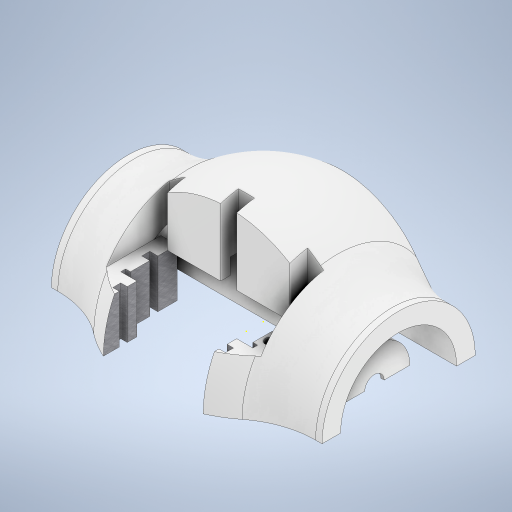
# Autodesk Inventor part: back moter middle lemon printing
Saved by Autodesk Inventor 2023 (Build 270158000, 158)
## iProperties
Created: 2022-10-08
Part Number: back moter middle lemon printing
Material: ABS プラスチック
Document SubType Name: Modeling
Designer: ellie
Density: 1.06 g/cm^3
Appearance: 積雪
Author: ellie
Autodesk Inventor part; units mm, degrees
ref_plane "YZ Plane" through (0, 0, 0) normal (1, 0, 0) x (0, 1, 0)
ref_plane "XZ Plane" through (0, 0, 0) normal (0, 1, 0) x (-1, 0, 0)
ref_plane "XY Plane" through (0, 0, 0) normal (0, 0, 1) x (1, 0, 0)
sketch "スケッチ1" plane through (0, 0, 0) normal (0, 1, 0) x (-1, 0, 0)
  circle A0 centre (0, 0) radius 37.5
  line L0 (0, 0) -> (0, -37.5)
  line L1 (0, 0) -> (0, 37.5)
  dimension "d0" = 75
  constraints: 4 end point, 2 point on circle, 2 vertical, 1 centre point, 1 coincident
  measures "d0" diameter of A0
revolve "回転1" add sketch "スケッチ1" angle 180 about axis through (0, 0, 0) along (0, 0, 1) picked at (-2.7815, -24.6866) contours L1 L0 A0
sketch "スケッチ5" plane through (0, 0, 0) normal (0, -1, 0) x (1, 0, 0)
  line L0 (-21, -21) -> (21, -21)
  line L1 (21, -21) -> (21, -9)
  line L2 (21, -9) -> (-21, -9)
  line L3 (-21, -9) -> (-21, -21)
  line L4 (-21, -11) -> (-21, -9)
  line L5 (0, 29.25) -> (-17.5, 29.25)
  line L6 (-17.5, 29.25) -> (-17.5, 26.75)
  line L7 (-17.5, 26.75) -> (0, 26.75)
  line L8 (0, 26.75) -> (0, 29.25)
  line L9 (0, 23.75) -> (-20.5, 23.75)
  line L10 (-20.5, 23.75) -> (-20.5, 22.25)
  line L11 (-20.5, 22.25) -> (0, 22.25)
  line L12 (0, 22.25) -> (0, 23.75)
  line L13 (0, 16.25) -> (-21.5, 16.25)
  line L14 (-21.5, 16.25) -> (-21.5, 13.75)
  line L15 (-21.5, 13.75) -> (0, 13.75)
  line L16 (0, 13.75) -> (0, 16.25)
  line L17 (0, 7.75) -> (-24, 7.75)
  line L18 (-24, 7.75) -> (-24, 5.25)
  line L19 (-24, 5.25) -> (0, 5.25)
  line L20 (0, 5.25) -> (0, 7.75)
  circle A0 centre (0, 0) radius 37.5 projected
  circle A1 centre (0, 0) radius 37.5 projected
  line L21 (0, 37.5) -> (0, -37.5)
  line L22 (37.5, 0) -> (-37.5, 0)
  line L23 (-33.5, 5.25) -> (-24, 5.25)
  line L24 (-24, 5.25) -> (-24, -5.25)
  line L25 (-24, -5.25) -> (-33.5, -5.25)
  line L26 (-33.5, -5.25) -> (-33.5, 5.25)
  line L27 (-24, -8.0262) -> (-24, 5.25)
  line L28 (-29, 23.775) -> (-29, -23.775)
  line L29 (-15.5, 29.25) -> (0, 29.25)
  line L30 (0, 29.25) -> (0, 37.5)
  line L31 (0, 37.5) -> (-15.5, 37.5)
  line L32 (-15.5, 37.5) -> (-15.5, 29.25)
  line L33 (-15.5, 26.75) -> (0, 26.75)
  line L34 (0, 26.75) -> (0, 23.75)
  line L35 (0, 23.75) -> (-15.5, 23.75)
  line L36 (-15.5, 23.75) -> (-15.5, 26.75)
  line L37 (-19, 16.25) -> (0, 16.25)
  line L38 (0, 16.25) -> (0, 22.25)
  line L39 (0, 22.25) -> (-19, 22.25)
  line L40 (-19, 22.25) -> (-19, 16.25)
  line L41 (-19, 13.75) -> (0, 13.75)
  line L42 (0, 13.75) -> (0, 7.75)
  line L43 (0, 7.75) -> (-19, 7.75)
  line L44 (-19, 7.75) -> (-19, 13.75)
  line L45 (-24, 0) -> (-40.9365, 0)
  line L46 (-24, 0) -> (-9.0837, 0)
  line L47 (-8.5, 5.25) -> (-24, 5.25)
  line L48 (-24, 5.25) -> (-24, -5.25)
  line L49 (-24, -5.25) -> (-8.5, -5.25)
  line L50 (-8.5, 5.25) -> (-24, -5.25) construction
  line L51 (-24, 5.25) -> (-8.5, -5.25) construction
  line L52 (-24, 7.25) -> (-34.5, 7.25)
  line L53 (-34.5, 7.25) -> (-34.5, -7.25)
  line L54 (-34.5, -7.25) -> (-24, -7.25)
  line L55 (-24, -7.25) -> (-24, 7.25)
  line L56 (-24, 7.25) -> (-34.5, -7.25) construction
  line L57 (-34.5, 7.25) -> (-24, -7.25) construction
  line L58 (-8.5, 5.25) -> (-1, 5.25)
  line L59 (-1, 5.25) -> (-1, -5.25)
  line L60 (-1, -5.25) -> (-8.5, -5.25)
  line L61 (-8.5, 5.25) -> (-1, -5.25) construction
  line L62 (-1, 5.25) -> (-8.5, -5.25) construction
  line L63 (-24, 5.25) -> (-29, 5.25)
  line L64 (-24, -5.25) -> (-29, -5.25)
  line L65 (-24, 7.25) -> (-29, 7.25)
  line L66 (-24, -7.25) -> (-29, -7.25)
  line L67 (28.3901, -24.5) -> (-28.3901, -24.5)
  line L68 (-8.5, 5.25) -> (-7.3, 5.25)
  line L69 (-7.3, -5.25) -> (-8.5, -5.25)
  line L70 (-4, 7.75) -> (-1, 7.75)
  line L71 (0, 23.75) -> (-4, 23.75)
  line L72 (-4, 22.25) -> (0, 22.25)
  line L73 (0, 22.25) -> (0, 23.75)
  line L74 (-7, 7.75) -> (-2, 7.75)
  line L75 (-1, 5.25) -> (-6.5, 5.25)
  point P0 (0, -21)
  point P1 (0, -9)
  point P2 (0, 28)
  point P3 (0, 23)
  point P4 (0, 15)
  point P5 (0, 6.5)
  point P6 (-21, -15)
  point P7 (-27, -0.5262)
  point P8 (-15.5, 25.25)
  point P9 (-15.5, 34.1467)
  point P10 (0, 29.25)
  point P11 (0, 26.75)
  point P12 (0, 13.75)
  point P13 (0, 16.25)
  point P14 (-29, 0)
  point P15 (-33.5, 0)
  point P16 (-24, 0)
  point P17 (-16.25, 0)
  point P18 (-29.25, 0)
  point P19 (-4.75, 0)
  point P20 (-27, 0.5)
  point P21 (-28, 0.4738)
  point P22 (-28, -11.5262)
  point P23 (-27, -11.5)
  point P24 (-24, 5.25)
  point P25 (-24, 5.25)
  point P26 (-24, 5.25)
  point P27 (-1, 0)
  point P28 (28.3901, -24.5)
  point P29 (-28.3901, -24.5)
  point P30 (0, 22.25)
  point P31 (0, 23.75)
  point P32 (-29, -7.25)
  point P33 (-29, 7.25)
  point P34 (-7.9, -5.25)
  point P35 (-7.9, 5.25)
  dimension "d12" = 42
  dimension "d13" = 12
  dimension "d23" = 17.5
  dimension "d24" = 2.5
  dimension "d27" = 20.5
  dimension "d28" = 1.5
  dimension "d30" = 21.5
  dimension "d31" = 2.5
  dimension "d33" = 2.5
  dimension "d88" = 0
  dimension "d89" = 0
  dimension "d90" = 16.5
  dimension "d92" = 21
  dimension "d97" = 9.5
  dimension "d98" = 10.5
  dimension "d113" = 29
  dimension "d122" = 15.5
  dimension "d124" = 3
  dimension "d125" = 15.5
  dimension "d126" = 6
  dimension "d127" = 6
  dimension "d128" = 19
  dimension "d129" = 19
  dimension "d161" = 14.5
  dimension "d162" = 10.5
  dimension "d164" = 10.5
  dimension "d170" = 24.5
  dimension "d326" = 23
  dimension "d327" = 10.5
  dimension "d329" = 15.5
  dimension "d330" = 34.5
  dimension "d357" = 8.25
  constraints: 150 end point, 28 parallel, 21 horizontal, 17 midpoint, 16 perpendicular, 16 point on line, 10 collinear, 1 tangent, 1 vertical, 20 other
  measures "d12" distance of L2.end L1.end
  measures "d13" distance of L1.end L0.end
  measures "d23" distance of L7.end L6.end
  measures "d24" distance of L6.end L5.end
  measures "d27" distance of L11.end L10.end
  measures "d28" distance of L10.end L9.end
  measures "d30" distance of L15.end L14.end
  measures "d31" distance of L14.end L13.end
  measures "d33" distance of L18.end L17.end
  measures "d89" distance from line of point (0, 0) L22
  measures "d90" distance from line of L0 point (0, -37.5)
  measures "d92" distance of the line from the sketch origin of L3
  measures "d97" distance of L24.end L25.end
  measures "d98" distance of L23.end L24.end
  measures "d113" distance of the line from the sketch origin of L28
  measures "d122" distance of the line from the sketch origin of L32
  measures "d124" distance of L33.end L34.end
  measures "d126" distance of L38.end L37.end
  measures "d127" distance of L41.end L42.end
  measures "d128" distance of the line from the sketch origin of L44
  measures "d129" distance of the line from the sketch origin of L40
  measures "d161" distance between parallel lines of L54 L52
  measures "d162" distance between parallel lines of L48 L53
  measures "d164" distance between parallel lines of L60 L58
  measures "d170" distance between parallel lines of L67 L22
  measures "d326" distance between parallel lines of L48 L59
  measures "d327" distance between parallel lines of L49 L47
  measures "d329" distance of L48.end L49.end
  measures "d330" distance of the line from the sketch origin of L53
  measures "d357" distance between parallel lines of L5 L31
extrude "GNSボード" cut sketch "スケッチ5" against normal blind 16 contours L8 L7 L6 L5
extrude "GNSボード止めるよう" cut sketch "スケッチ5" against normal blind 15 contours L21 L5 L32 A0 | L21 L9 L36 L7
extrude "アルミ板１" cut sketch "スケッチ5" against normal blind 20 contours L11 L10 L9 L12
extrude "メイン基板" cut sketch "スケッチ5" against normal blind 21 contours L15 L14 L13 L16
extrude "メイン止めるよう" cut sketch "スケッチ5" against normal blind 15 contours L17 L44 L15 L21 | L13 L40 L11 L21
extrude "アルミ板２" cut sketch "スケッチ5" against normal blind 20 contours L19 L18 L17 L20
extrude "電池ボックス入れ" cut sketch "スケッチ5" against normal blind 13 contours L3 L2 L21 L0 | L21 L2 L1 L0
extrude "side ut" cut sketch "スケッチ5" against normal blind 100 contours A0 L22 L53 L54 L28 | A0 L28 L52 L53 L22 | L54 L53 L22 L26 L25 L28 | L53 L52 L28 L23 L26 L22 | L25 L26 L22 L28 | L22 L26 L23 L28
extrude "motor case" add sketch "スケッチ5" against normal blind 7 contours L54 L53 L22 L26 L25 L28 | L28 L25 L27 L54 | L24 L25 L28 L22 | L22 L28 L23 L24 | L53 L52 L28 L23 L26 L22 | L25 L26 L22 L28 | L22 L26 L23 L28 | L23 L28 L52 L18
extrude "bottom cut" cut sketch "スケッチ5" against normal blind 90 contours L67 A0 L21 | L21 A0 L67
extrude "motor" cut sketch "スケッチ5" against normal blind 6 contours L59 L60 L49 L24 L22 | L22 L24 L19 L59 | L24 L25 L28 L22 | L22 L28 L23 L24 | L25 L26 L22 L28 | L22 L26 L23 L28
sketch "スケッチ27" plane through (-34.5, 0, -7.25) normal (-1, 0, 0) x (0, 0, 1)
  line L0 (14.5, 0) -> (0, 0) projected
  circle A0 centre (7.25, 0) radius 3
  point P0 (7.25, 0)
  dimension "d198" = 6
  constraints: 1 centre point, 1 midpoint
  measures "d198" diameter of A0
extrude "moter shaft" cut sketch "スケッチ27" against normal blind 27
mirror "ミラー13" about plane through (0, 0, 0) normal (1, 0, 0) of "メイン止めるよう", "メイン基板", "アルミ板１", "GNSボード止めるよう", "GNSボード", "アルミ板２", "motor", "motor case", "moter shaft", "電池ボックス入れ", "side ut"
ref_plane "作業平面5" through (-17.5, 17.5, 26.75) normal (0, -1, 0) x (1, 0, 0)
ref_plane "作業平面6" through (21, 13, -9) normal (0, 0, -1) x (1, 0, 0)
ref_plane "作業平面7" through (29, 35, 7.25) normal (0, -1, 0) x (1, 0, 0)
sketch "スケッチ41" plane through (-17.5, 0, 26.75) normal (0, -1, 0) x (1, 0, 0)
  line L0 (-17, -23.75) -> (-16, -23.75) projected
  line L1 (-16, -23.75) -> (-16, -21.5) projected
  line L2 (-16, -21.5) -> (-6.5, -21.5) projected
  line L3 (-6.5, -21.5) -> (-6.5, -19) projected
  line L4 (-6.5, -19) -> (-1.5, -19) projected
  line L5 (-1.5, -19) -> (-1.5, -13) projected
  line L6 (-1.5, -13) -> (-4, -13) projected
  line L7 (-4, -13) -> (-4, -10.5) projected
  line L8 (-4, -10.5) -> (-1.5, -10.5) projected
  line L9 (-1.5, -10.5) -> (-1.5, -4.5) projected
  line L10 (-1.5, -4.5) -> (-3, -4.5) projected
  line L11 (-3, -4.5) -> (-3, -3) projected
  line L12 (-3, -3) -> (2, -3) projected
  line L13 (2, -3) -> (2, 0) projected
  line L14 (2, 0) -> (0, 0) projected
  line L15 (0, 0) -> (0, 2.5) projected
  line L16 (0, 2.5) -> (2, 2.5) projected
  line L17 (2, 2.5) -> (2, 7.3967) projected
  arc A0 (2, 7.3967) -> (-11.5, -2.975) centre (17.5, -26.75) ccw projected
  line L18 (-11.5, -2.975) -> (-11.5, -19.5) projected
  line L19 (-11.5, -19.5) -> (-17, -19.5) projected
  line L20 (-17, -19.5) -> (-17, -23.75) projected
  line L21 (-1.5, -19) -> (-1.5, -13) projected
  line L22 (-4, -10.5) -> (-4, -13) projected
  line L23 (0, 2.5) -> (0, 0) projected
  circle A1 centre (-4, -0.5) radius 2.4
  dimension "d252" = 4.8
  dimension "d253" = 4
  dimension "d254" = 2.5
  constraints: 1 centre point
  measures "d252" diameter of A1
  measures "d253" distance from line of A1.centre L15
  measures "d254" distance from line of A1.centre L12
extrude "top lock 10mm" cut sketch "スケッチ41" against normal blind 3 contours A1
mirror "ミラー15" about plane through (0, 0, 0) normal (1, 0, 0) of "top lock 10mm"
sketch "スケッチ42" plane through (-34.5, 0, -7.25) normal (0, -1, 0) x (1, 0, 0)
  circle A0 centre (9.5, -14) radius 2.4
  line L0 (13.5, -13.75) -> (13.5, -1.75) projected
  line L1 (33.5, 2) -> (1, 2) projected
  point P0 (34.5, 7.25)
  point P1 (10, 2)
  point P2 (7.8183, 2)
  point P3 (12.1817, 2)
  dimension "d257" = 4
  dimension "d258" = 4.8
  dimension "d259" = 16
  constraints: 1 centre point
  measures "d257" distance from line of A0.centre L0
  measures "d258" diameter of A0
  measures "d259" distance from line of A0.centre L1
extrude "bottom lock" cut sketch "スケッチ42" against normal blind 3
mirror "ミラー16" about plane through (0, 0, 0) normal (1, 0, 0) of "bottom lock"
ref_plane "作業平面8" through (-17.5, 15, 26.75) normal (0, -1, 0) x (1, 0, 0)
sketch "スケッチ45" plane through (-17.5, 15, 26.75) normal (0, -1, 0) x (1, 0, 0)
  circle A0 centre (-4, -0.5) radius 2.4 projected
  line L0 (-17, -23.75) -> (-16, -23.75) projected
  line L1 (-16, -23.75) -> (-16, -21.5) projected
  line L2 (-16, -21.5) -> (-6.5, -21.5) projected
  line L3 (-6.5, -21.5) -> (-6.5, -19) projected
  line L4 (-6.5, -19) -> (-1.5, -19) projected
  line L5 (-1.5, -19) -> (-1.5, -13) projected
  line L6 (-1.5, -13) -> (-4, -13) projected
  line L7 (-4, -13) -> (-4, -10.5) projected
  line L8 (-4, -10.5) -> (-1.5, -10.5) projected
  line L9 (-1.5, -10.5) -> (-1.5, -4.5) projected
  line L10 (-1.5, -4.5) -> (-3, -4.5) projected
  line L11 (-3, -4.5) -> (-3, -3) projected
  line L12 (-3, -3) -> (2, -3) projected
  line L13 (2, -3) -> (2, 0) projected
  line L14 (2, 0) -> (0, 0) projected
  line L15 (0, 0) -> (0, 2.5) projected
  line L16 (0, 2.5) -> (2, 2.5) projected
  line L17 (2, 2.5) -> (2, 7.3967) projected
  arc A1 (2, 7.3967) -> (-11.5, -2.975) centre (17.5, -26.75) ccw projected
  line L18 (-11.5, -2.975) -> (-11.5, -19.5) projected
  line L19 (-11.5, -19.5) -> (-17, -19.5) projected
  line L20 (-17, -19.5) -> (-17, -23.75) projected
  arc A2 (33, 3.9257) -> (2, 3.9257) centre (17.5, -26.75) ccw projected
  line L21 (2, 2.5) -> (2, 3.9257) projected
  line L22 (33, 2.5) -> (2, 2.5) projected
  line L23 (33, 2.5) -> (33, 3.9257) projected
  circle A3 centre (39, -0.5) radius 2.4 projected
  line L24 (51, -23.75) -> (52, -23.75) projected
  line L25 (52, -19.5) -> (52, -23.75) projected
  line L26 (46.5, -19.5) -> (52, -19.5) projected
  line L27 (46.5, -19.5) -> (46.5, -2.975) projected
  arc A4 (46.5, -2.975) -> (33, 7.3967) centre (17.5, -26.75) ccw projected
  line L28 (33, 7.3967) -> (33, 2.5) projected
  line L29 (33, 2.5) -> (35, 2.5) projected
  line L30 (35, 2.5) -> (35, 0) projected
  line L31 (35, 0) -> (33, 0) projected
  line L32 (33, 0) -> (33, -3) projected
  line L33 (33, -3) -> (38, -3) projected
  line L34 (38, -3) -> (38, -4.5) projected
  line L35 (38, -4.5) -> (36.5, -4.5) projected
  line L36 (36.5, -4.5) -> (36.5, -10.5) projected
  line L37 (36.5, -10.5) -> (39, -10.5) projected
  line L38 (39, -10.5) -> (39, -13) projected
  line L39 (39, -13) -> (36.5, -13) projected
  line L40 (36.5, -13) -> (36.5, -19) projected
  line L41 (36.5, -19) -> (41.5, -19) projected
  line L42 (41.5, -19) -> (41.5, -21.5) projected
  line L43 (41.5, -21.5) -> (51, -21.5) projected
  line L44 (51, -21.5) -> (51, -23.75) projected
  circle A5 centre (39, -0.5) radius 2.4 projected
  arc A6 (-17, -23.75) -> (-17, -23.75) centre (-4, -0.5) ccw projected
  line L45 (35, 0) -> (0, 0) projected
  line L46 (35, 0) -> (35, 2.3017) projected
  line L47 (34.6665, 2.5) -> (0.3335, 2.5) projected
  line L48 (0, 0) -> (0, 2.3017) projected
  line L49 (33, -3) -> (2, -3) projected
  line L50 (33, -3) -> (33, 0) projected
  line L51 (2, 0) -> (33, 0) projected
  line L52 (2, -3) -> (2, 0) projected
  line L53 (-1.5, -4.5) -> (36.5, -4.5) projected
  arc A7 (51, -23.75) -> (51, -23.75) centre (39, -0.5) ccw projected
  line L54 (36.5, -10.5) -> (-1.5, -10.5) projected
  line L55 (36.5, -10.5) -> (36.5, -4.5) projected
  line L56 (-1.5, -4.5) -> (36.5, -4.5) projected
  line L57 (-1.5, -10.5) -> (-1.5, -4.5) projected
  line L58 (-1.5, -13) -> (36.5, -13) projected
  line L59 (36.5, -19) -> (-1.5, -19) projected
  line L60 (36.5, -19) -> (36.5, -13) projected
  line L61 (-1.5, -13) -> (36.5, -13) projected
  line L62 (-1.5, -19) -> (-1.5, -13) projected
  line L63 (41.5, -21.5) -> (-6.5, -21.5) projected
  line L64 (41.5, -21.5) -> (41.5, -19) projected
  line L65 (41.5, -19) -> (-6.5, -19) projected
  line L66 (-6.5, -21.5) -> (-6.5, -19) projected
  line L67 (-6.5, -21.5) -> (16.5, -21.5) projected
  line L68 (-16, -21.5) -> (-6.5, -21.5) projected
  line L69 (-16, -32) -> (-16, -21.5) projected
  line L70 (16.5, -32) -> (-16, -32) projected
  circle A8 centre (42.5, -48) radius 2.4 projected
  circle A9 centre (-7.5, -48) radius 2.4 projected
  line L71 (18.5, -32) -> (18.5, -21.5) projected
  line L72 (18.5, -21.5) -> (16.5, -21.5) projected
  line L73 (16.5, -21.5) -> (16.5, -32) projected
  line L74 (-6.5, -21.5) -> (-6.5, -19) projected
  line L75 (-16, -32) -> (-16, -29.75) projected
  line L76 (-16, -29.75) -> (-17, -29.75) projected
  line L77 (-17, -29.75) -> (-17, -34) projected
  line L78 (-17, -34) -> (-11.5, -34) projected
  line L79 (-11.5, -34) -> (-11.5, -50.525) projected
  arc A10 (-11.5, -50.525) -> (-10.8901, -51.25) centre (17.5, -26.75) ccw projected
  line L80 (-10.8901, -51.25) -> (45.8901, -51.25) projected
  arc A11 (45.8901, -51.25) -> (46.5, -50.525) centre (17.5, -26.75) ccw projected
  line L81 (46.5, -50.525) -> (46.5, -34) projected
  line L82 (52, -34) -> (46.5, -34) projected
  line L83 (52, -29.75) -> (52, -34) projected
  line L84 (52, -29.75) -> (51, -29.75) projected
  line L85 (51, -29.75) -> (51, -32) projected
  line L86 (41.5, -19) -> (41.5, -21.5) projected
  line L87 (-3.5, -35.75) -> (38.5, -35.75) projected
  line L88 (38.5, -35.75) -> (38.5, -47.75) projected
  line L89 (38.5, -47.75) -> (-3.5, -47.75) projected
  line L90 (-3.5, -47.75) -> (-3.5, -35.75) projected
  line L91 (-6.5, -16) -> (41.5, -16)
  line L92 (41.5, -16) -> (41.5, 7.6193)
  line L93 (41.5, 7.6193) -> (-6.5, 7.6193)
  line L94 (-6.5, 7.6193) -> (-6.5, -16)
  line L95 (16.5, -21.5) -> (16.5, -32) projected
  line L96 (-17, -23.75) -> (-16, -23.75) projected
  line L97 (-16, -23.75) -> (-16, -21.5) projected
  line L98 (-16, -21.5) -> (-6.5, -21.5) projected
  line L99 (-6.5, -19) -> (-1.5, -19) projected
  line L100 (-1.5, -19) -> (-1.5, -13) projected
  line L101 (-1.5, -13) -> (-4, -13) projected
  line L102 (-4, -13) -> (-4, -10.5) projected
  line L103 (-4, -10.5) -> (-1.5, -10.5) projected
  line L104 (-1.5, -10.5) -> (-1.5, -4.5) projected
  line L105 (-1.5, -4.5) -> (-3, -4.5) projected
  line L106 (-3, -4.5) -> (-3, -3) projected
  line L107 (-3, -3) -> (2, -3) projected
  line L108 (2, -3) -> (2, 0) projected
  line L109 (2, 0) -> (0, 0) projected
  line L110 (0, 0) -> (0, 2.5) projected
  line L111 (0, 2.5) -> (2, 2.5) projected
  line L112 (2, 2.5) -> (2, 7.3967) projected
  line L113 (-11.5, -2.975) -> (-11.5, -19.5) projected
  line L114 (-11.5, -19.5) -> (-17, -19.5) projected
  line L115 (-17, -19.5) -> (-17, -23.75) projected
  line L116 (16.5, -32) -> (-16, -32) projected
  line L117 (51, -32) -> (18.5, -32) projected
  line L118 (51, -23.75) -> (52, -23.75) projected
  line L119 (52, -19.5) -> (52, -23.75) projected
  line L120 (46.5, -19.5) -> (52, -19.5) projected
  line L121 (46.5, -19.5) -> (46.5, -2.975) projected
  line L122 (33, 7.3967) -> (33, 2.5) projected
  line L123 (33, 2.5) -> (35, 2.5) projected
  line L124 (35, 2.5) -> (35, 0) projected
  line L125 (35, 0) -> (33, 0) projected
  line L126 (33, 0) -> (33, -3) projected
  line L127 (33, -3) -> (38, -3) projected
  line L128 (38, -3) -> (38, -4.5) projected
  line L129 (38, -4.5) -> (36.5, -4.5) projected
  line L130 (36.5, -4.5) -> (36.5, -10.5) projected
  line L131 (36.5, -10.5) -> (39, -10.5) projected
  line L132 (39, -10.5) -> (39, -13) projected
  line L133 (39, -13) -> (36.5, -13) projected
  line L134 (36.5, -13) -> (36.5, -19) projected
  line L135 (36.5, -19) -> (41.5, -19) projected
  line L136 (41.5, -21.5) -> (51, -21.5) projected
  line L137 (51, -21.5) -> (51, -23.75) projected
  arc A12 (2, 7.3967) -> (-11.5, -2.975) centre (17.5, -26.75) ccw projected
  arc A13 (46.5, -2.975) -> (33, 7.3967) centre (17.5, -26.75) ccw projected
  arc A14 (0.3335, 2.5) -> (0, 2.3017) centre (17.5, -26.75) ccw projected
  arc A15 (35, 2.3017) -> (34.6665, 2.5) centre (17.5, -26.75) ccw projected
  arc A16 (45.8901, -51.25) -> (46.5, -50.525) centre (17.5, -26.75) ccw projected
  arc A17 (-11.5, -50.525) -> (-10.8901, -51.25) centre (17.5, -26.75) ccw projected
  circle A18 centre (-4, -0.5) radius 2.4 projected
  circle A19 centre (39, -0.5) radius 2.4 projected
  line L138 (52, -29.75) -> (51, -29.75) projected
  line L139 (51, -32) -> (18.5, -32) projected
  line L140 (18.5, -32) -> (18.5, -21.5) projected
  line L141 (18.5, -21.5) -> (16.5, -21.5) projected
  line L142 (16.5, -21.5) -> (16.5, -32) projected
  line L143 (16.5, -32) -> (-16, -32) projected
  line L144 (-17, -23.75) -> (-16, -23.75) projected
  line L145 (-16, -29.75) -> (-17, -29.75) projected
  line L146 (-16, -32) -> (-16, -29.75) projected
  line L147 (-17, -29.75) -> (-17, -34) projected
  line L148 (-17, -34) -> (-11.5, -34) projected
  line L149 (-11.5, -34) -> (-11.5, -50.525) projected
  arc A20 (-11.5, -50.525) -> (-10.8901, -51.25) centre (17.5, -26.75) ccw projected
  line L150 (-10.8901, -51.25) -> (45.8901, -51.25) projected
  line L151 (46.5, -50.525) -> (46.5, -34) projected
  line L152 (52, -34) -> (46.5, -34) projected
  line L153 (52, -29.75) -> (52, -34) projected
  line L154 (51, -29.75) -> (51, -32) projected
  line L155 (52, -29.75) -> (51, -29.75) projected
  line L156 (51, -23.75) -> (52, -23.75) projected
  line L157 (51, -32) -> (18.5, -32) projected
  line L158 (18.5, -32) -> (18.5, -21.5) projected
  line L159 (18.5, -21.5) -> (16.5, -21.5) projected
  line L160 (16.5, -21.5) -> (16.5, -32) projected
  line L161 (16.5, -32) -> (-16, -32) projected
  line L162 (-16, -29.75) -> (-17, -29.75) projected
  line L163 (-16, -32) -> (-16, -29.75) projected
  line L164 (-17, -29.75) -> (-17, -34) projected
  line L165 (-17, -34) -> (-11.5, -34) projected
  line L166 (-11.5, -34) -> (-11.5, -50.525) projected
  line L167 (-10.8901, -51.25) -> (45.8901, -51.25) projected
  arc A21 (45.8901, -51.25) -> (46.5, -50.525) centre (17.5, -26.75) ccw projected
  line L168 (46.5, -50.525) -> (46.5, -34) projected
  line L169 (52, -34) -> (46.5, -34) projected
  line L170 (52, -29.75) -> (52, -34) projected
  line L171 (51, -29.75) -> (51, -32) projected
  line L172 (-16, -23.75) -> (-16, -21.5) projected
  line L173 (-16, -21.5) -> (-6.5, -21.5) projected
  line L174 (-6.5, -21.5) -> (-6.5, -19) projected
  line L175 (-6.5, -19) -> (-1.5, -19) projected
  line L176 (-1.5, -19) -> (-1.5, -13) projected
  line L177 (-1.5, -13) -> (-4, -13) projected
  line L178 (-4, -13) -> (-4, -10.5) projected
  line L179 (-4, -10.5) -> (-1.5, -10.5) projected
  line L180 (-1.5, -10.5) -> (-1.5, -4.5) projected
  line L181 (-1.5, -4.5) -> (-3, -4.5) projected
  line L182 (-3, -4.5) -> (-3, -3) projected
  line L183 (-3, -3) -> (2, -3) projected
  line L184 (2, -3) -> (2, 0) projected
  line L185 (2, 0) -> (0, 0) projected
  line L186 (0, 0) -> (0, 2.5) projected
  line L187 (0, 2.5) -> (2, 2.5) projected
  line L188 (2, 2.5) -> (2, 7.3967) projected
  arc A22 (2, 7.3967) -> (-11.5, -2.975) centre (17.5, -26.75) ccw projected
  line L189 (-11.5, -2.975) -> (-11.5, -19.5) projected
  line L190 (-11.5, -19.5) -> (-17, -19.5) projected
  line L191 (-17, -19.5) -> (-17, -23.75) projected
  line L192 (52, -19.5) -> (52, -23.75) projected
  line L193 (46.5, -19.5) -> (52, -19.5) projected
  line L194 (46.5, -19.5) -> (46.5, -2.975) projected
  arc A23 (46.5, -2.975) -> (33, 7.3967) centre (17.5, -26.75) ccw projected
  line L195 (33, 7.3967) -> (33, 2.5) projected
  line L196 (33, 2.5) -> (35, 2.5) projected
  line L197 (35, 2.5) -> (35, 0) projected
  line L198 (35, 0) -> (33, 0) projected
  line L199 (33, 0) -> (33, -3) projected
  line L200 (33, -3) -> (38, -3) projected
  line L201 (38, -3) -> (38, -4.5) projected
  line L202 (38, -4.5) -> (36.5, -4.5) projected
  line L203 (36.5, -4.5) -> (36.5, -10.5) projected
  line L204 (36.5, -10.5) -> (39, -10.5) projected
  line L205 (39, -10.5) -> (39, -13) projected
  line L206 (39, -13) -> (36.5, -13) projected
  line L207 (36.5, -13) -> (36.5, -19) projected
  line L208 (36.5, -19) -> (41.5, -19) projected
  line L209 (41.5, -19) -> (41.5, -21.5) projected
  line L210 (41.5, -21.5) -> (51, -21.5) projected
  line L211 (51, -21.5) -> (51, -23.75) projected
  dimension "d269" = 3
  constraints: 8 end point, 2 collinear, 2 parallel, 1 horizontal, 1 perpendicular, 1 tangent, 2 other
  measures "d269" distance between parallel lines of L91 L65
extrude "back cut" cut sketch "スケッチ45" against normal blind 25 contours A0 | L93 L92 A4 L28 A2 A6 | A6 A2 L93 | L93 A2 A7 | A7 A2 L17 A1 L94 L93 | A6 L22 A7 A2 | A2 L23 L22 A6 | A7 L22 L17 A2 | A1 L17 L16 L15 L14 L13 L12 L11 L10 L9 L8 L7 L6 L5 L91 L94 | L28 A4 L92 L91 L40 L39 L38 L37 L36 L35 L34 L33 L32 L31 L30 L29 L23 | A6 L45 A7 L22 | L22 L29 A15 L30 L31 L45 A6 | A7 L45 L14 L15 A14 L16 L22 | L91 L5 L58 A7 A6 | A6 A7 L91 | L45 L32 L49 A6 | A6 L49 A7 L45 | A7 L49 L13 L45 | A7 L58 A6 | A6 L58 L40 L91 A7 | L29 L30 A15 | A14 L15 L16 | A7 L53 L10 L11 L12 L49 | L49 A6 L53 A7 | L58 A7 L54 A6 | A6 L54 L37 L38 L39 L58 | L58 L6 L7 L8 L54 A7 | L49 L33 L34 L35 L53 A6 | A7 L54 L9 L53 | L53 A6 L54 A7 | A6 L53 L36 L54 | A3
sketch "スケッチ52" plane through (21, 0, -9) normal (0, 0, -1) x (-1, 0, 0)
  line L0 (42, 0) -> (0, 0) projected
  line L1 (42, 0) -> (42, 13) projected
  line L2 (42, 13) -> (0, 13) projected
  line L3 (0, 0) -> (0, 13) projected
  line L4 (22, 6) -> (54.5, 6) projected
  line L5 (54.5, 0) -> (54.5, 6) projected
  line L6 (22, 0) -> (54.5, 0) projected
  line L7 (22, 0) -> (54.5, 0) projected
  line L8 (22, 0) -> (22, 6) projected
  line L9 (22, 6) -> (54.5, 6) projected
  line L10 (20, 6) -> (-12.5, 6) projected
  line L11 (20, 0) -> (20, 6) projected
  line L12 (-12.5, 0) -> (20, 0) projected
  line L13 (-12.5, 0) -> (20, 0) projected
  line L14 (-12.5, 0) -> (-12.5, 6) projected
  line L15 (20, 6) -> (-12.5, 6) projected
  line L16 (29, 10) -> (39, 10)
  line L17 (39, 10) -> (39, 16)
  line L18 (39, 16) -> (29, 16)
  line L19 (29, 16) -> (29, 10)
  line L20 (20, 0) -> (20, 6) projected
  line L21 (-12.5, 0) -> (-12.5, 6) projected
  line L22 (54.5, 0) -> (54.5, 6) projected
  line L23 (22, 0) -> (22, 6) projected
  point P0 (21, 0)
  dimension "d293" = 3
  dimension "d294" = 10
  dimension "d295" = 4
  constraints: 8 end point, 2 parallel, 1 horizontal, 1 perpendicular, 1 other
  measures "d293" distance between parallel lines of L1 L17
  measures "d294" distance between parallel lines of L17 L19
  measures "d295" distance between parallel lines of L16 L4
extrude "押し出し54" cut sketch "スケッチ52" against normal up to surface (16.75 mm away) contours L17 L16 L19 L2 | L2 L19 L18 L17
sketch "スケッチ53" plane through (0, 13, 0) normal (0, -1, 0) x (1, 0, 0)
  line L0 (-8, -9) -> (-8, 5.25) projected
  line L1 (-18, -9) -> (-8, -9) projected
  line L2 (-18, -9) -> (-18, 5.25) projected
  line L3 (-18, -9) -> (-18, 5.25) projected
  line L4 (-18, -9) -> (-18, 5.25) projected
  line L5 (-24, 10.75) -> (24, 10.75) projected
  line L6 (24, 10.75) -> (24, 24.6018) projected
  line L7 (15.5, 30.6757) -> (15.5, 34.1467) projected
  arc A0 (29, 23.775) -> (15.5, 34.1467) centre (0, 0) ccw projected
  line L8 (29, 23.775) -> (29, -23.775) projected
  line L9 (28.3901, -24.5) -> (-28.3901, -24.5) projected
  arc A1 (-29, -23.775) -> (-28.3901, -24.5) centre (0, 0) ccw projected
  line L10 (-29, -23.775) -> (-29, 23.775) projected
  line L11 (-15.5, 34.1467) -> (-15.5, 30.6757) projected
  line L12 (-24, 24.6018) -> (-24, 10.75) projected
  line L13 (-18, -9) -> (-8, -9)
  line L14 (-8, -9) -> (-8, -15)
  line L15 (-8, -15) -> (-18, -15)
  line L16 (-18, -15) -> (-18, -9)
  arc A2 (28.3901, -24.5) -> (29, -23.775) centre (0, 0) ccw projected
  arc A3 (-15.5, 34.1467) -> (-29, 23.775) centre (0, 0) ccw projected
  arc A4 (-15.5, 30.6757) -> (-24, 24.6018) centre (0, 0) ccw projected
  arc A5 (24, 24.6018) -> (15.5, 30.6757) centre (0, 0) ccw projected
  point P0 (-18, -9)
  point P1 (-8, -9)
  dimension "d298" = 6
  constraints: 8 end point, 3 collinear, 2 parallel, 1 horizontal, 1 perpendicular
  measures "d298" distance between parallel lines of L15 L1
extrude "押し出し55" cut sketch "スケッチ53" against normal up to surface (3 mm away) contours L1 L14 L15 L16
sketch "スケッチ54" plane through (-24, 15, 10.75) normal (0, 0, 1) x (1, 0, 0)
  line L0 (43, 0) -> (48, 0) projected
  line L1 (48, 0) -> (43, 0)
  line L2 (43, 0) -> (43, 22.5)
  line L3 (43, 22.5) -> (48, 22.5)
  line L4 (48, 22.5) -> (48, 0)
  line L5 (0, 0) -> (5, 0) projected
  line L6 (0, 0) -> (5, 0)
  line L7 (5, 0) -> (5, 22.5)
  line L8 (5, 22.5) -> (0, 22.5)
  line L9 (0, 22.5) -> (0, 0)
  line L10 (24, -15) -> (24, 22.5)
  arc A0 (53, 8.775) -> (-5, 8.775) centre (24, -15) ccw projected
  line L11 (26.5, 0) -> (21.5, 0)
  line L12 (21.5, 0) -> (21.5, 22.5)
  line L13 (21.5, 22.5) -> (26.5, 22.5)
  line L14 (26.5, 22.5) -> (26.5, 0)
  line L15 (43, 0) -> (5, 0) projected
  arc A1 (48, 11.7336) -> (0, 11.7336) centre (24, -15) ccw projected
  line L16 (0, 0) -> (0, 11.7336) projected
  line L17 (0, 0) -> (5, 0) projected
  line L18 (43, 0) -> (5, 0) projected
  line L19 (43, 0) -> (48, 0) projected
  line L20 (48, 0) -> (48, 11.7336) projected
  line L21 (39.5, 0) -> (39.5, -15) projected
  line L22 (39.5, -15) -> (53, -15) projected
  line L23 (53, -15) -> (53, -15) projected
  arc A2 (52.3901, -15) -> (-4.3901, -15) centre (24, -15) ccw projected
  line L24 (-4.3901, -15) -> (-5, -15) projected
  line L25 (-5, -15) -> (-5, -15) projected
  line L26 (8.5, -15) -> (8.5, 0) projected
  line L27 (0, 0) -> (0, 11.7336) projected
  arc A3 (48, 11.7336) -> (0, 11.7336) centre (24, -15) ccw projected
  line L28 (48, 11.7336) -> (48, 0) projected
  line L29 (53, -15) -> (52.3901, -15) projected
  line L30 (-5, -15) -> (8.5, -15) projected
  line L31 (8.5, 0) -> (0, 0) projected
  line L32 (48, 0) -> (39.5, 0) projected
  point P0 (21.5, 0)
  point P1 (21.5, 22.4166)
  point P2 (5, 17.3303)
  point P3 (43, 17.3303)
  point P4 (26.5, 22.4166)
  point P5 (43, 15.4908)
  point P6 (26.5, 20.839)
  point P7 (21.5, 20.839)
  point P8 (5, 15.4908)
  point P9 (0, 11.7336)
  point P10 (48, 13.8141)
  point P11 (0, 13.8141)
  dimension "d301" = 5
  dimension "d302" = 5
  dimension "d303" = 2.5
  dimension "d304" = 5
  constraints: 26 end point, 6 parallel, 3 horizontal, 3 perpendicular, 3 tangent, 1 collinear, 1 point on circle, 1 vertical
  measures "d301" distance of L2.end L3.end
  measures "d302" distance of L8.end L7.end
  measures "d303" distance between parallel lines of L14 L10
  measures "d304" distance between parallel lines of L14 L12
extrude "押し出し56" cut sketch "スケッチ54" against normal up to surface (5.5 mm away) contours L2 A2 L4 L0 | L2 A1 L4 A2 | L2 A0 L4 A1 | A2 L10 A1 L14 | L14 L11 L10 A2 | L2 L3 L4 A0 | A1 L10 A0 L14 | A2 L12 A1 L10 | L10 L11 L12 A2 | A0 L13 L14 | A1 L12 A0 L10 | A0 L12 L13 | A2 L9 A1 L7 | L7 L5 L9 A2 | A1 L9 A0 L7
sketch "スケッチ55" plane through (-29, 0, 7.25) normal (-1, 0, 0) x (0, 0, 1)
  arc A0 (16.525, 0) -> (-31.025, 0) centre (-7.25, 0) ccw projected
  line L0 (-14.5, 7) -> (0, 7) projected
  line L1 (0, 0) -> (0, 7) projected
  line L2 (-14.5, 0) -> (-14.5, 7) projected
  arc A1 (-4.25, 0) -> (-10.25, 0) centre (-7.25, 0) ccw projected
  line L3 (-14.5, 0) -> (0, 0) projected
  line L4 (16.525, 0) -> (0, 0) projected
  line L5 (-2, 0) -> (-12.5, 0) projected
  circle A2 centre (-7.25, 0) radius 11
  line L6 (-14.5, 0) -> (-31.025, 0) projected
  point P0 (-31, 8)
  point P1 (-31, 0)
  point P2 (3.75, 0)
  point P3 (-18, 0)
  point P4 (-18.25, 0)
  dimension "d309" = 22
  constraints: 1 centre point, 1 coincident
  measures "d309" diameter of A2
extrude "モーター受け円形" add sketch "スケッチ55" along normal up to surface (5.5 mm away) contours L4 L1 L0 L2 L6 A2
sketch "スケッチ57" plane through (-29, 0, 0) normal (-1, 0, 0) x (0, 0, 1)
  circle A0 centre (0, 0) radius 16
  circle A1 centre (0, 0) radius 18
  line L0 (23.775, 0) -> (11, 0) projected
  line L1 (-3, 0) -> (-11, 0) projected
  line L2 (11, 0) -> (3, 0) projected
  line L3 (5.25, 0) -> (-5.25, 0) projected
  arc A2 (3, 0) -> (-3, 0) centre (0, 0) ccw projected
  line L4 (11, 0) -> (3, 0) projected
  arc A3 (11, 0) -> (-11, 0) centre (0, 0) ccw projected
  line L5 (-3, 0) -> (-11, 0) projected
  arc A4 (11, 0) -> (-11, 0) centre (0, 0) ccw projected
  line L6 (23.775, 0) -> (11, 0) projected
  arc A5 (23.775, 0) -> (-23.775, 0) centre (0, 0) ccw projected
  line L7 (-11, 0) -> (-23.775, 0) projected
  point P0 (-16, 0)
  point P1 (-11, 0)
  point P2 (11, 0)
  point P3 (16, 0)
  point P4 (-18, 0)
  point P5 (18, 0)
  dimension "d314" = 32
  dimension "d315" = 36
  constraints: 2 centre point, 2 coincident
  measures "d314" diameter of A0
  measures "d315" diameter of A1
extrude "押し出し59" cut sketch "スケッチ57" against normal blind 5 contours L0 A3 L7 A0
extrude "押し出し60" cut sketch "スケッチ57" against normal blind 5 contours A0 L7 A1 L0 picked at (-17.159, 1.4359)
mirror "ミラー17" about plane through (0, 0, 0) normal (1, 0, 0) of "モーター受け円形", "押し出し59", "押し出し60"
ref_plane "作業平面9" through (42, 0, 0) normal (1, 0, 0) x (0, 0, -1)
sketch "スケッチ59" plane through (42, 0, 0) normal (1, 0, 0) x (0, 0, -1)
  circle A0 centre (0, 0) radius 23
  arc A1 (18, 0) -> (-18, 0) centre (0, 0) ccw projected
  circle A2 centre (0, 0) radius 18
  line L0 (-23.775, 0) -> (-34.1467, 0) projected
  line L1 (-18, 0) -> (-23.775, 0) projected
  line L2 (-11, 0) -> (-18, 0) projected
  line L3 (-11, 0) -> (-3, 0) projected
  line L4 (5.25, 0) -> (-5.25, 0) projected
  line L5 (3, 0) -> (11, 0) projected
  line L6 (18, 0) -> (11, 0) projected
  line L7 (23.775, 0) -> (18, 0) projected
  arc A3 (23.775, 0) -> (-23.775, 0) centre (0, 0) ccw projected
  line L8 (-23.775, 0) -> (23.775, 0)
  point P0 (0, 0)
  point P1 (17.6, 0)
  dimension "d321" = 46
  constraints: 2 centre point, 2 coincident, 2 end point, 1 concentric
  measures "d321" diameter of A0
extrude "押し出し61" add sketch "スケッチ59" against normal up to surface (13 mm away) contours L7 A1 L1 A0 | A0 L1 A3 L7
sketch "スケッチ60" plane through (24, 0, 5.25) normal (0, -1, 0) x (1, 0, 0)
  point P0 (-24, -5.25)
fillet "面フィレット1" radius 27.7 1 edges at (29, 23.775, 0)
mirror "ミラー18" about plane through (0, 0, 0) normal (1, 0, 0) of "面フィレット1", "押し出し61"
ref_plane "作業平面11" through (0, 13, 0) normal (0, -1, 0) x (1, 0, 0)
sketch "スケッチ61" plane through (0, 13, 0) normal (0, -1, 0) x (1, 0, 0)
  point P0 (0, 0)
sketch "スケッチ62" plane through (-24, 0, 5.25) normal (0, 0, -1) x (-1, 0, 0)
  point P0 (-24, 0)
sketch "スケッチ63" plane through (-24, 0, 5.25) normal (0, 0, -1) x (-1, 0, 0)
  line L0 (10.5, 11) -> (10.5, 0) projected
  line L1 (0, 0) -> (10.5, 0) projected
  line L2 (-21.5, 20) -> (-21.5, 37.0464) projected
  arc A0 (-21.5, 37.0464) -> (-26.5, 37.0464) centre (-24, 0) ccw projected
  arc A1 (-26.5, 37.0464) -> (-43, 31.9012) centre (-24, 0) ccw projected
  arc A2 (-43, 31.9012) -> (-47.016, 29.1368) centre (-24, 0) ccw projected
  line L3 (-66, 23.1881) -> (-64.0171, 23.1881) projected
  line L4 (-66, 17.2174) -> (-66, 23.1881) projected
  line L5 (-48, 17.2174) -> (-66, 17.2174) projected
  line L6 (-48, 9.6663) -> (-48, 17.2174) projected
  line L7 (-48, 9.6663) -> (-48, 6) projected
  line L8 (-25, 6) -> (-48, 6) projected
  line L9 (-25, 0) -> (-25, 6) projected
  line L10 (-23, 0) -> (-25, 0) projected
  line L11 (-23, 6) -> (-23, 0) projected
  line L12 (0, 6) -> (-23, 6) projected
  line L13 (0, 6) -> (0, 9.6663) projected
  line L14 (0, 9.6663) -> (10.5, 9.6663) projected
  line L15 (10.5, 9.6663) -> (10.5, 0) projected
  line L16 (10.5, 0) -> (9.5, 0) projected
  line L17 (9.5, 0) -> (0, 0) projected
  line L18 (0, 0) -> (0, 6) projected
  line L19 (9.5, 6) -> (0, 6) projected
  line L20 (9.5, 0) -> (9.5, 6) projected
  line L21 (-5, 20) -> (-21.5, 20) projected
  line L22 (-5, 31.9012) -> (-5, 20) projected
  arc A3 (-0.984, 29.1368) -> (-5, 31.9012) centre (-24, 0) ccw projected
  line L23 (16.0171, 23.1881) -> (18, 23.1881) projected
  line L24 (18, 23.1881) -> (18, 17.2174) projected
  line L25 (18, 17.2174) -> (0, 17.2174) projected
  line L26 (0, 17.2174) -> (0, 9.6663) projected
  arc A4 (-5, 31.9012) -> (-21.5, 37.0464) centre (-24, 0) ccw projected
  line L27 (-26.5, 37.0464) -> (-26.5, 20) projected
  line L28 (-26.5, 20) -> (-43, 20) projected
  line L29 (-43, 20) -> (-43, 31.9012) projected
  line L30 (-48, 28.3941) -> (-48, 17.2174) projected
  line L31 (-58.5, 9.6663) -> (-48, 9.6663) projected
  line L32 (-58.5, 0) -> (-58.5, 9.6663) projected
  line L33 (-57.5, 0) -> (-58.5, 0) projected
  line L34 (-57.5, 6) -> (-57.5, 0) projected
  line L35 (-48, 6) -> (-57.5, 6) projected
  line L36 (-48, 6) -> (-48, 0) projected
  line L37 (-48, 0) -> (-57.5, 0) projected
  line L38 (0, 17.2174) -> (0, 28.3941) projected
  line L39 (-6, 16) -> (-16, 16) projected
  line L40 (-16, 16) -> (-16, 10) projected
  line L41 (-16, 10) -> (-6, 10) projected
  line L42 (-6, 10) -> (-6, 16) projected
  line L43 (4.5, 0) -> (2.5, 0)
  line L44 (2.5, 0) -> (2.5, 6)
  line L45 (2.5, 6) -> (4.5, 6)
  line L46 (4.5, 6) -> (4.5, 0)
  point P0 (4.5, 0)
  point P1 (4.5, 6)
  point P2 (2.5, 6)
  point P3 (2.5, 0)
  dimension "d334" = 6
  dimension "d335" = 8
  dimension "d336" = 6
  constraints: 8 end point, 2 parallel, 1 collinear, 1 horizontal, 1 perpendicular, 4 other
  measures "d334" distance between parallel lines of L46 L0
  measures "d335" distance between parallel lines of L44 L0
  measures "d336" distance between parallel lines of L45 L43
extrude "押し出し62" add sketch "スケッチ63" along normal blind 3 contours L1 L44 L19 L46
mirror "ミラー19" about plane through (0, 0, 0) normal (1, 0, 0) of "押し出し62"
sketch "スケッチ64" plane through (-33.5, 0, -5.25) normal (0, -1, 0) x (1, 0, 0)
  line L0 (32.5, 10.5) -> (32.5, 0) projected
  line L1 (34.5, 0) -> (34.5, 10.5) projected
  line L2 (57.5, -5.75) -> (68, -5.75) projected
  line L3 (68, 2.25) -> (68, -5.75) projected
  line L4 (68, 2.25) -> (67, 2.25) projected
  line L5 (67, 2.25) -> (67, 0) projected
  line L6 (67, 0) -> (34.5, 0) projected
  line L7 (34.5, 0) -> (34.5, 10.5) projected
  line L8 (34.5, 10.5) -> (32.5, 10.5) projected
  line L9 (32.5, 10.5) -> (32.5, 0) projected
  line L10 (32.5, 0) -> (0, 0) projected
  line L11 (0, 0) -> (0, 2.25) projected
  line L12 (0, 2.25) -> (-1, 2.25) projected
  line L13 (-1, 2.25) -> (-1, -5.75) projected
  line L14 (-1, -5.75) -> (9.5, -5.75) projected
  line L15 (9.5, -5.75) -> (9.5, -12.75) projected
  line L16 (-8.5, -12.75) -> (9.5, -12.75) projected
  line L17 (-8.5, -12.75) -> (-8.5, -18.525) projected
  line L18 (-8.5, -18.525) -> (-6.5171, -18.525) projected
  line L19 (-0.221, -19.25) -> (67.221, -19.25) projected
  line L20 (75.5, -18.525) -> (73.5171, -18.525) projected
  line L21 (75.5, -12.75) -> (75.5, -18.525) projected
  line L22 (75.5, -12.75) -> (57.5, -12.75) projected
  line L23 (57.5, -12.75) -> (57.5, -5.75) projected
  line L24 (12.5, -3.75) -> (54.5, -3.75) projected
  line L25 (54.5, -3.75) -> (54.5, -15.75) projected
  line L26 (54.5, -15.75) -> (12.5, -15.75) projected
  line L27 (12.5, -15.75) -> (12.5, -3.75) projected
  circle A0 centre (8.5, -16) radius 2.4 projected
  circle A1 centre (58.5, -16) radius 2.4 projected
  line L28 (9.5, 10.5) -> (32.5, 10.5) projected
  line L29 (32.5, 10.5) -> (34.5, 10.5)
  line L30 (34.5, 10.5) -> (34.5, 0)
  line L31 (34.5, 0) -> (32.5, 0)
  line L32 (32.5, 0) -> (32.5, 10.5)
  point P0 (33.5, 5.25)
  point P1 (32.5, 0)
  point P2 (32.5, 10.5)
  constraints: 8 end point, 2 parallel, 1 horizontal, 1 perpendicular, 2 other
extrude "押し出し63" cut sketch "スケッチ64" against normal up to surface (6 mm away) contours L8 L1 L31 L0
sketch "スケッチ65" plane through (33.721, 0, -24.5) normal (0, 0, -1) x (-1, 0, 0)
  line L0 (67.4421, 0) -> (0, 0) projected
  arc A0 (56.737, 16.6213) -> (10.7051, 16.6213) centre (33.721, 0) ccw projected
  circle A1 centre (28.721, 23) radius 2.4
  circle A2 centre (38.721, 23) radius 2.4
  line L1 (33.721, 0) -> (33.721, 28.3901)
  dimension "d341" = 4.8
  dimension "d342" = 4.8
  dimension "d343" = 10
  dimension "d344" = 23
  dimension "d345" = 23
  dimension "d347" = 5
  constraints: 2 centre point, 2 end point, 1 point on circle, 2 other
  measures "d341" diameter of A1
  measures "d342" diameter of A2
  measures "d343" distance of A2.centre A1.centre
  measures "d344" distance from line of A1.centre L0
  measures "d345" distance from line of L0 A2.centre
  measures "d347" distance from line of L1 A1.centre
extrude "押し出し64" cut sketch "スケッチ65" against normal blind 3
sketch "スケッチ66" plane through (-17.5, 15, 26.75) normal (0, 1, 0) x (1, 0, 0)
  circle A0 centre (39, 7.5733) radius 1.65
  line L0 (36.5, 10.5) -> (36.5, 4.5) projected
  line L1 (38, 4.5) -> (36.5, 4.5) projected
  line L2 (41.5, 16.8001) -> (41.5, 2.0764) projected
  line L3 (40.516, 21.5) -> (36.5, 21.5) projected
  point P0 (17.5, 26.75)
  point P1 (36.5, 7.5)
  dimension "d350" = 3.3
  dimension "d355" = 2.5
  dimension "d356" = 13.9267
  constraints: 1 centre point, 1 midpoint
  measures "d350" diameter of A0
  measures "d355" distance from line of A0.centre L2
  measures "d356" distance from line of A0.centre L3
extrude "押し出し65" cut sketch "スケッチ66" against normal blind 3
